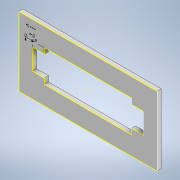
# Autodesk Inventor part: EngravingJig
Saved by Autodesk Inventor 2022 (Build 260153000, 153)
## iProperties
Created: 2021-02-01
Part Number: EngravingJig
Material: Generic
Document SubType Name: Modeling
Designer: Viktor
Density: 1 g/cm^3
Appearance: Default
Author: Viktor
Autodesk Inventor part; units mm, degrees
ref_plane "YZ Plane" through (0, 0, 0) normal (1, 0, 0) x (0, 1, 0)
ref_plane "XZ Plane" through (0, 0, 0) normal (0, 1, 0) x (-1, 0, 0)
ref_plane "XY Plane" through (0, 0, 0) normal (0, 0, 1) x (1, 0, 0)
sketch "Sketch1" plane through (0, 0, 0) normal (0, 0, 1) x (1, 0, 0)
  line L0 (-100, -50) -> (100, -50)
  line L1 (100, -50) -> (100, 50)
  line L2 (100, 50) -> (-100, 50)
  line L3 (-100, 50) -> (-100, -50)
  line L4 (-100, -50) -> (100, 50) construction
  line L5 (100, -50) -> (-100, 50) construction
  line L6 (-63, -23) -> (63, -23)
  line L7 (63, -23) -> (63, 23)
  line L8 (63, 23) -> (-63, 23)
  line L9 (-63, 23) -> (-63, -23)
  line L10 (-63, -23) -> (63, 23) construction
  line L11 (63, -23) -> (-63, 23) construction
  point P0 (0, 0)
  dimension "d0" = 200
  dimension "d1" = 100
  dimension "d2" = 126
  dimension "d3" = 46
  constraints: 24 end point, 4 midpoint, 4 parallel, 2 horizontal, 2 perpendicular
  measures "d0" distance of L1.end L2.end
  measures "d1" distance of L2.end L0.start
  measures "d2" distance between parallel lines of L7 L9
  measures "d3" distance between parallel lines of L8 L6
extrude "Extrusion1" add sketch "Sketch1" along normal blind 6
sketch "Sketch2" plane through (0, 0, 6) normal (0, 0, 1) x (1, 0, 0)
  line L0 (-80, -15) -> (80, -15)
  line L1 (80, -15) -> (80, 15)
  line L2 (80, 15) -> (-80, 15)
  line L3 (-80, 15) -> (-80, -15)
  line L4 (-80, -15) -> (80, 15) construction
  line L5 (80, -15) -> (-80, 15) construction
  point P0 (0, 0)
  dimension "d6" = 160
  dimension "d7" = 30
  constraints: 12 end point, 2 midpoint, 2 parallel, 1 horizontal, 1 perpendicular
  measures "d6" distance between parallel lines of L1 L3
  measures "d7" distance between parallel lines of L0 L2
extrude "Extrusion2" cut sketch "Sketch2" against normal through all
sketch "Sketch3" plane through (0, 0, 6) normal (0, 0, 1) x (1, 0, 0)
  line L0 (-90.4385, 41.5009) -> (-72.2585, 41.5009) construction
  line L1 (-72.2585, 41.5009) -> (-72.2585, 36.1823) construction
  line L2 (-72.2585, 36.1823) -> (-90.4385, 36.1823) construction
  line L3 (-90.4385, 36.1823) -> (-90.4385, 41.5009) construction
  circle A0 centre (-80, 23) radius 0.25
  line L4 (-80, -15) -> (-80, 15) projected
  line L5 (-63, 23) -> (63, 23) projected
  line L6 (100, -50) -> (100, 50) projected
  line L7 (100, 50) -> (-100, 50) projected
  line L8 (-100, 50) -> (-100, -50) projected
  line L9 (-100, -50) -> (100, -50) projected
  line L10 (63, 15) -> (80, 15) projected
  line L11 (80, 15) -> (80, -15) projected
  line L12 (80, -15) -> (63, -15) projected
  line L13 (63, -15) -> (63, -23) projected
  line L14 (63, -23) -> (-63, -23) projected
  line L15 (-63, -23) -> (-63, -15) projected
  line L16 (-63, -15) -> (-80, -15) projected
  line L17 (-80, -15) -> (-80, 15) projected
  line L18 (-80, 15) -> (-63, 15) projected
  line L19 (-63, 15) -> (-63, 23) projected
  line L20 (-63, 23) -> (63, 23) projected
  line L21 (63, 23) -> (63, 15) projected
  point P0 (0, 0)
  dimension "d10" = 0
  dimension "d11" = 0
  dimension "d12" = 0.5
  constraints: 1 centre point, 2 other
  measures "d10" distance from line of L4 A0.centre
  measures "d11" distance from line of L5 A0.centre
  measures "d12" diameter of A0
extrude "Extrusion3" cut sketch "Sketch3" against normal through all contours A0
body "Solid1"
